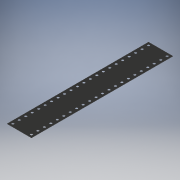
# Autodesk Inventor part: Foam NPS 8
Saved by Autodesk Inventor 2019 (Build 230136000, 136)
## iProperties
Created: 2016-08-30
Part Number: Foam NPS 8
Material: Rubber, Silicone
Document SubType Name: Modeling
Designer: IEUser
Density: 1.25 g/cm^3
Appearance: Rubber - Black
Author: IEUser
Autodesk Inventor part; units mm, degrees
ref_plane "YZ Plane" through (0, 0, 0) normal (1, 0, 0) x (0, 1, 0)
ref_plane "XZ Plane" through (0, 0, 0) normal (0, 1, 0) x (-1, 0, 0)
ref_plane "XY Plane" through (0, 0, 0) normal (0, 0, 1) x (1, 0, 0)
sketch "Foam Scheme" plane through (0, 0, 0) normal (0, 1, 0) x (-1, 0, 0)
  line L0 (547, -94) -> (-547, -94)
  line L1 (-547, -94) -> (-547, 94)
  line L2 (-547, 94) -> (547, 94)
  line L3 (547, 94) -> (547, -94)
  circle A0 centre (525, -72) radius 9.5
  circle A1 centre (475, -72) radius 9.5
  circle A2 centre (425, -72) radius 9.5
  circle A3 centre (375, -72) radius 9.5
  circle A4 centre (325, -72) radius 9.5
  circle A5 centre (275, -72) radius 9.5
  circle A6 centre (225, -72) radius 9.5
  circle A7 centre (175, -72) radius 9.5
  circle A8 centre (125, -72) radius 9.5
  circle A9 centre (75, -72) radius 9.5
  circle A10 centre (25, -72) radius 9.5
  circle A11 centre (-25, -72) radius 9.5
  circle A12 centre (-75, -72) radius 9.5
  circle A13 centre (-125, -72) radius 9.5
  circle A14 centre (-175, -72) radius 9.5
  circle A15 centre (-225, -72) radius 9.5
  circle A16 centre (-275, -72) radius 9.5
  circle A17 centre (-325, -72) radius 9.5
  circle A18 centre (525, 72) radius 9.5
  circle A19 centre (475, 72) radius 9.5
  circle A20 centre (425, 72) radius 9.5
  circle A21 centre (375, 72) radius 9.5
  circle A22 centre (325, 72) radius 9.5
  circle A23 centre (275, 72) radius 9.5
  circle A24 centre (225, 72) radius 9.5
  circle A25 centre (175, 72) radius 9.5
  circle A26 centre (125, 72) radius 9.5
  circle A27 centre (75, 72) radius 9.5
  circle A28 centre (25, 72) radius 9.5
  circle A29 centre (-25, 72) radius 9.5
  circle A30 centre (-75, 72) radius 9.5
  circle A31 centre (-125, 72) radius 9.5
  circle A32 centre (-175, 72) radius 9.5
  circle A33 centre (-225, 72) radius 9.5
  circle A34 centre (-275, 72) radius 9.5
  circle A35 centre (-325, 72) radius 9.5
  circle A36 centre (-375, -72) radius 9.5
  circle A37 centre (-375, 72) radius 9.5
  circle A38 centre (-425, -72) radius 9.5
  circle A39 centre (-425, 72) radius 9.5
  circle A40 centre (-475, -72) radius 9.5
  circle A41 centre (-475, 72) radius 9.5
  circle A42 centre (-525, -72) radius 9.5
  circle A43 centre (-525, 72) radius 9.5
  point P0 (0, 0)
  dimension "d0" = 1094
  dimension "d1" = 547
  dimension "d2" = 188
  dimension "d3" = 94
  dimension "d4" = 19
  dimension "d5" = 22
  dimension "d6" = 22
  dimension "d9" = 50
  dimension "d12" = 144
  constraints: 44 centre point, 8 end point, 2 horizontal, 2 parallel, 1 perpendicular, 1 vertical, 86 other
  measures "d0" distance of L0.start L0.end
  measures "d1" distance from line of point (0, 0) L3
  measures "d2" distance of L2.end L0.start
  measures "d3" distance from line of point (0, 0) L0
  measures "d4" diameter of A0
  measures "d5" distance from line of L3 A0.centre
  measures "d6" distance from line of L0 A0.centre
  measures "d9" distance of A0.centre A1.centre
  measures "d12" distance of A0.centre A18.centre
extrude "Foam Body" add sketch "Foam Scheme" along normal blind 1.5
equation "\"d1\" = 0.5 * d0"
equation "\"d3\" = 0.5 * d2"
body "Solid2"
